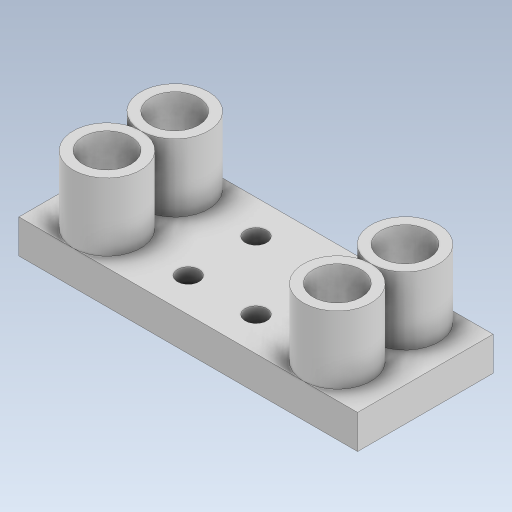
# Autodesk Inventor part: Fix Double Bracket Lifter
Saved by Autodesk Inventor 2023.5 (Build 275446000, 446)
## iProperties
Created: 2025-10-01
Part Number: Fix Double Bracket Lifter
Material: Generic
Document SubType Name: Modeling
Designer: Guntur
Density: 1 g/cm^3
Appearance: Default
Author: Guntur
## iProperties of the stored document Fix Double Bracket Lifter_3DPrint.ipt
Created: 2025-10-13
Part Number: Fix Double Bracket Lifter_3DPrint
Material: Generic
Document SubType Name: Modeling
Designer: Guntur
Density: 1 g/cm^3
Appearance: Default
Author: Guntur
Autodesk Inventor part; units mm, degrees
ref_plane "YZ Plane" through (0, 0, 0) normal (1, 0, 0) x (0, 1, 0)
ref_plane "XZ Plane" through (0, 0, 0) normal (0, 1, 0) x (-1, 0, 0)
ref_plane "XY Plane" through (0, 0, 0) normal (0, 0, 1) x (1, 0, 0)
sketch "Sketch1" plane through (0, 0, 0) normal (0, 1, 0) x (-1, 0, 0)
  line L0 (25, 10) -> (-25, 10)
  line L1 (-25, 10) -> (-25, -10)
  line L2 (-25, -10) -> (25, -10)
  line L3 (25, -10) -> (25, 10)
  line L4 (25, 10) -> (-25, -10) construction
  line L5 (-25, 10) -> (25, -10) construction
  circle A0 centre (-17, 5) radius 3.55
  line L6 (32, 0) -> (-42, 0) construction
  line L7 (0, 26) -> (0, -35) construction
  circle A1 centre (-5, 5) radius 1.6
  circle A2 centre (-17, -5) radius 3.55
  circle A3 centre (-5, -5) radius 1.6
  circle A4 centre (17, 5) radius 3.55
  circle A5 centre (5, 5) radius 1.6
  circle A6 centre (5, -5) radius 1.6
  circle A7 centre (17, -5) radius 3.55
  circle A8 centre (-17, -5) radius 5
  circle A9 centre (-17, 5) radius 5
  circle A10 centre (17, 5) radius 5
  circle A11 centre (17, -5) radius 5
  point P0 (0, 0)
  point P1 (17, 10)
  point P2 (17, 0)
  point P3 (17, -10)
  point P4 (-17, 10)
  point P5 (-17, 0)
  point P6 (-17, -10)
  dimension "d0" = 50
  dimension "d1" = 20
  dimension "d2" = 7.1
  dimension "d3" = 5
  dimension "d4" = 3.2
  dimension "d5" = 12
  dimension "d6" = 10
  dimension "d7" = 10
  dimension "d8" = 10
  dimension "d9" = 10
  constraints: 16 end point, 12 centre point, 6 symmetric about line, 4 coincident, 2 horizontal, 2 midpoint, 2 parallel, 1 perpendicular, 1 vertical, 6 other
  measures "d0" distance of L2.end L1.end
  measures "d1" distance of L1.end L0.end
  measures "d2" diameter of A0
  measures "d3" distance from line of L0 A0.centre
  measures "d4" diameter of A1
  measures "d5" distance of A0.centre A1.centre
  measures "d6" diameter of A8
  measures "d7" diameter of A9
  measures "d8" diameter of A10
  measures "d9" diameter of A11
extrude "Extrusion1" add sketch "Sketch1" along normal blind 5 contours L3 L2 A11 A10 L0 | A10 A11 L2 A8 A9 L0 | A9 A8 L2 L1 L0
extrude "Extrusion2" add sketch "Sketch1" along normal blind 15 contours A10 | A9 | A11 | A8
body "Solid1"
